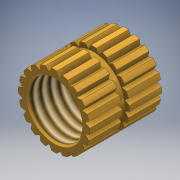
# Autodesk Inventor part: knurled_insert_M3_4
Saved by Autodesk Inventor 2016 (Build 200138000, 138)
## iProperties
Created: 2016-09-25
Part Number: knurled_insert_M3_4
Material: Brass, Soft Yellow
Document SubType Name: Modeling
Designer: Luke
Density: 8.47 g/cm^3
Appearance: Brass - Satin
Author: Luke
Autodesk Inventor part; units mm, degrees
ref_plane "YZ Plane" through (0, 0, 0) normal (1, 0, 0) x (0, 1, 0)
ref_plane "XZ Plane" through (0, 0, 0) normal (0, 1, 0) x (-1, 0, 0)
ref_plane "XY Plane" through (0, 0, 0) normal (0, 0, 1) x (1, 0, 0)
sketch "Sketch1" plane through (0, 0, 0) normal (0, 1, 0) x (-1, 0, 0)
  circle A0 centre (0, 0) radius 1.5
  circle A1 centre (0, 0) radius 1.75
  dimension "d0" = 3
  dimension "d1" = 3.5
  constraints: 2 centre point, 2 coincident
  measures "d0" diameter of A0
  measures "d1" diameter of A1
extrude "Extrusion1" add sketch "Sketch1" along normal blind 4
sketch "Sketch2" plane through (0, 4, 0) normal (0, 1, 0) x (1, 0, 0)
  circle A0 centre (0, 0) radius 1.5 projected
  circle A1 centre (0, 0) radius 1.75 projected
  circle A2 centre (0, 0) radius 2
  dimension "d4" = 4
  constraints: 1 centre point, 1 coincident
  measures "d4" diameter of A2
extrude "Extrusion2" add sketch "Sketch2" against normal blind 1.8 contours A2
ref_plane "Work Plane1" through (0, 2, 0) normal (0, -1, 0) x (1, 0, 0)
mirror "Mirror1" about plane through (0, 2, 0) normal (0, -1, 0) of "Extrusion2"
thread "Thread1" size "M3x0.5" class "6H" standard "ISO Metric profile" full length
chamfer "Chamfer1" distance 0.1 angle 45 2 edges at (1.5, 0, 0) (1.5, 4, 0)
sketch "Sketch3" plane through (0, 0, 0) normal (0, -1, 0) x (1, 0, 0)
  circle A0 centre (0, 0) radius 2 projected
  circle A1 centre (0, 0) radius 1.6 projected
  line L0 (0, 0) -> (0.3129, -1.9754) construction
  line L1 (0, 0) -> (-0.3129, -1.9754) construction
  circle A2 centre (0, 0) radius 2 construction
  line L2 (0, 0) -> (0, -2) construction
  circle A3 centre (0, 0) radius 1.75 construction
  line L3 (0.2738, -1.7285) -> (0.15, -1.9944)
  line L4 (-0.2738, -1.7285) -> (-0.15, -1.9944)
  line L5 (0, 2.8) -> (0, -2.8) projected
  line L6 (0.2738, -1.7285) -> (0.3129, -1.9754)
  line L7 (-0.2738, -1.7285) -> (-0.3129, -1.9754)
  dimension "d12" = 18
  dimension "d13" = 3.5
  dimension "d14" = 0.3
  constraints: 14 end point, 11 point on circle, 3 collinear, 2 point on line, 1 centre point, 1 coincident, 2 other
  measures "d12" angle of L1 L0
  measures "d13" diameter of A3
  measures "d14" distance of L4.end L3.end
extrude "Extrusion3" cut sketch "Sketch3" against normal up to surface (4 mm away) contours L7 L4 A0 | L3 L6 A0
pattern_circular "Circular Pattern1" count 20 over 360 about axis through (0, -10, 0) along (0, 1, 0) of "Extrusion3"
body "Solid1"
